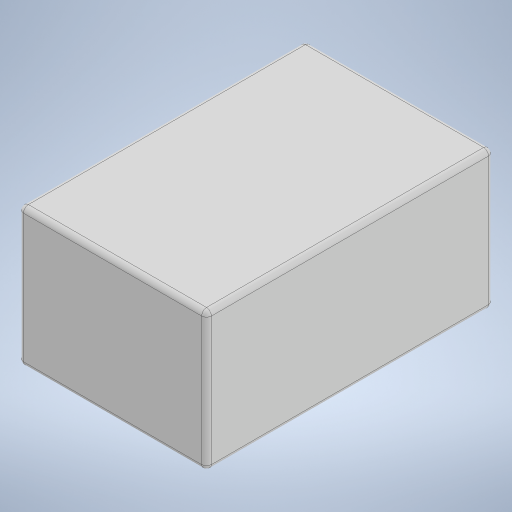
# Autodesk Inventor part: box elektronik
Saved by Autodesk Inventor 2023 (Build 270158000, 158)
## iProperties
Created: 2023-09-20
Part Number: box elektronik
Material: Generic
Document SubType Name: Modeling
Designer: sigit
Density: 1 g/cm^3
Appearance: Default
Author: sigit
Autodesk Inventor part; units mm, degrees
ref_plane "YZ Plane" through (0, 0, 0) normal (1, 0, 0) x (0, 1, 0)
ref_plane "XZ Plane" through (0, 0, 0) normal (0, 1, 0) x (-1, 0, 0)
ref_plane "XY Plane" through (0, 0, 0) normal (0, 0, 1) x (1, 0, 0)
sketch "Sketch1" plane through (0, 0, 0) normal (0, 1, 0) x (-1, 0, 0)
  line L0 (0, 0) -> (19, 0)
  line L1 (19, 0) -> (19, -29)
  line L2 (19, -29) -> (0, -29)
  line L3 (0, -29) -> (0, 0)
  dimension "d0" = 19
  dimension "d1" = 29
  constraints: 8 end point, 2 parallel, 1 horizontal, 1 perpendicular
  measures "d0" distance of L1.end L2.end
  measures "d1" distance of L0.end L1.end
extrude "Extrusion1" add sketch "Sketch1" along normal blind 14
fillet "Fillet1" radius 0.5 12 edges at (-9.5, 14, -29) (-9.5, 0, -29) (-19, 7, -29) (-19, 14, -14.5) (-19, 0, -14.5) (-19, 7, 0) (-9.5, 14, 0) (-9.5, 0, 0) (0, 7, 0) (0, 14, -14.5) (0, 7, -29) (0, 0, -14.5)
body "Solid1"
